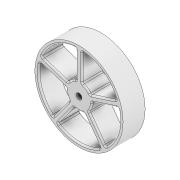
# Autodesk Inventor part: wheel
Saved by Autodesk Inventor 2020 (Build 240168000, 168)
## iProperties
Created: 2020-09-08
Part Number: wheel
Material: ABS 플라스틱
Document SubType Name: Modeling
Designer: 이호석
Mass: 133.383 g
Surface Area: 414.379 cm^2
Volume: 125.833 cm^3
Density: 1.06 g/cm^3
Appearance: 매끄러움 - 흰색
Author: 이호석
Autodesk Inventor part; units mm, degrees
ref_plane "YZ Plane" through (0, 0, 0) normal (1, 0, 0) x (0, 1, 0)
ref_plane "XZ Plane" through (0, 0, 0) normal (0, 1, 0) x (-1, 0, 0)
ref_plane "XY Plane" through (0, 0, 0) normal (0, 0, 1) x (1, 0, 0)
sketch "스케치1" plane through (0, 0, 0) normal (0, 0, 1) x (1, 0, 0)
  circle A0 centre (0, 0) radius 72.5
  circle A1 centre (0, 0) radius 55
  circle A2 centre (0, 0) radius 4
  circle A3 centre (0, 0) radius 17.5
  line L0 (-4, 17.0367) -> (-4, 54.8544)
  line L1 (4, 17.0367) -> (4, 54.8544)
  line L2 (-17.439, 1.4604) -> (-53.4057, 13.1467)
  line L3 (-14.9668, 9.0689) -> (-50.9335, 20.7552)
  line L4 (-6.7779, -16.1341) -> (-29.0065, -46.7292)
  line L5 (-13.25, -11.4319) -> (-35.4786, -42.027)
  line L6 (13.25, -11.4319) -> (35.4786, -42.027)
  line L7 (6.7779, -16.1341) -> (29.0065, -46.7292)
  line L8 (14.9668, 9.0689) -> (50.9335, 20.7552)
  line L9 (17.439, 1.4604) -> (53.4057, 13.1467)
  circle A4 centre (0, 0) radius 60
  point P0 (53.4057, 13.1467)
  dimension "d6" = 360
  dimension "d8" = 120
  constraints: 20 end point, 5 centre point, 5 coincident, 4 point on circle, 1 tangent, 1 vertical, 31 other
  measures "d8" diameter of A4
extrude "돌출1" add sketch "스케치1" along normal blind 30 contours L9 A3 L8 A1 | A1 L7 A3 L6 | A3 | L1 A3 L0 A1 | A1 L5 A3 L4 | L3 A3 L2 A1 | A4
fillet "모깎기1" radius 2 60 edges at (-10.2862, 14.1578, 30) (-10.2862, 14.1578, 0) (-14.9668, 9.0689, 15) (-32.9502, 14.912, 30) (-32.9502, 14.912, 0) (-16.6435, -5.4078, 30) (-16.6435, -5.4078, 0) (-52.3081, -16.9959, 30) (-52.3081, -16.9959, 0) (-13.25, -11.4319, 15) (13.25, -11.4319, 15) (-24.3643, -26.7294, 30) (-24.3643, -26.7294, 0) (-35.4786, -42.027, 15) (-17.8922, -31.4317, 30) (17.8922, -31.4317, 30) (17.8922, -31.4317, 0) (-17.8922, -31.4317, 0) (-6.7779, -16.1341, 15) (6.7779, -16.1341, 15) (0, -17.5, 30) (0, -17.5, 0) (-29.0065, -46.7292, 15) (0, -55, 30) (0, -55, 0) (-17.439, 1.4604, 15) (-4, 17.0367, 15) (-35.4223, 7.3036, 30) (-35.4223, 7.3036, 0) (-4, 35.9455, 30) (-4, 35.9455, 0) (-4, 54.8544, 15) (-32.3282, 44.4959, 0) (-32.3282, 44.4959, 30) (-50.9335, 20.7552, 15) (29.0065, -46.7292, 15) (-53.4057, 13.1467, 15) (17.439, 1.4604, 15) (35.4223, 7.3036, 30) (35.4223, 7.3036, 0) (53.4057, 13.1467, 15) (32.9502, 14.912, 30) (32.9502, 14.912, 0) (14.9668, 9.0689, 15) (10.2862, 14.1578, 0) (4, 17.0367, 15) (10.2862, 14.1578, 30) (4, 54.8544, 15) (4, 35.9455, 0) (4, 35.9455, 30) (50.9335, 20.7552, 15) (32.3282, 44.4959, 30) (32.3282, 44.4959, 0) (16.6435, -5.4078, 30) (16.6435, -5.4078, 0) (24.3643, -26.7294, 30) (24.3643, -26.7294, 0) (52.3081, -16.9959, 30) (52.3081, -16.9959, 0) (35.4786, -42.027, 15)
